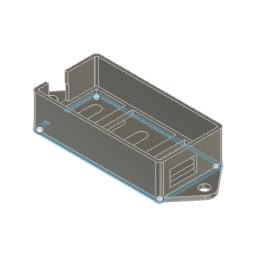
PSU case v4 (Autodesk Fusion 360 design; units mm, degrees)
Autodesk Fusion 360 part; units mm, degrees
sketch "Sketch1" plane through (0, 0, 0) normal (0, 0, 1) x (1, 0, 0) in component "card"
  line L0 (0, 0) -> (63, 0)
  line L1 (63, 0) -> (63, 30)
  line L2 (63, 30) -> (0, 30)
  line L3 (0, 30) -> (0, 0)
  line L4 (1, 29) -> (8.5, 29)
  line L5 (8.5, 29) -> (8.5, 19)
  line L6 (8.5, 19) -> (1, 19)
  line L7 (1, 19) -> (1, 29)
  line L8 (1, 6) -> (14.5, 6)
  line L9 (14.5, 6) -> (14.5, 15)
  line L10 (14.5, 15) -> (1, 15)
  line L11 (1, 15) -> (1, 6)
  line L12 (62, 29) -> (54.5, 29)
  line L13 (54.5, 29) -> (54.5, 19)
  line L14 (54.5, 19) -> (62, 19)
  line L15 (62, 19) -> (62, 29)
  line L16 (62, 4) -> (52, 4)
  line L17 (52, 4) -> (52, 17)
  line L18 (52, 17) -> (62, 17)
  line L19 (62, 17) -> (62, 4)
  dimension "d1" = 63
  dimension "d2" = 30
  dimension "d3" = 7.5
  dimension "d4" = 10
  dimension "d5" = 13.5
  dimension "d6" = 9
  dimension "d7" = 7.5
  dimension "d8" = 10
  dimension "d9" = 10
  dimension "d10" = 13
  constraint horizontal L0
  constraint vertical L1
  constraint horizontal L2
  constraint vertical L3
  constraint coincident L0.start L3.end
  constraint horizontal L4
  constraint vertical L5
  constraint horizontal L6
  constraint vertical L7
  constraint horizontal L8
  constraint vertical L9
  constraint horizontal L10
  constraint vertical L11
  constraint horizontal L12
  constraint vertical L13
  constraint horizontal L14
  constraint vertical L15
  constraint horizontal L16
  constraint vertical L17
  constraint horizontal L18
  constraint vertical L19
  measures "d1" distance of L0.start L0.end
  measures "d2" distance of L0.start L2.end
  measures "d3" distance of L4.start L4.end
  measures "d4" distance of L4.start L6.end
  measures "d5" distance of L8.start L8.end
  measures "d6" distance of L8.start L10.end
  measures "d7" distance of L12.start L12.end
  measures "d8" distance of L12.start L14.end
  measures "d9" distance of L16.start L16.end
  measures "d10" distance of L16.start L18.end
sketch "pcb support 0,4.5" plane through (0, 0, 0) normal (0, 0, 1) x (1, 0, 0) in component "bottom"
  line L0 (62.5, 29) -> (62.5, 1)
  line L1 (1, 1) -> (1, 29)
  line L2 (20, 1) -> (20, 29)
  line L3 (16.0721, 29) -> (16.0721, 1)
  line L4 (42.6148, 29) -> (42.6148, 1)
  line L5 (47, 1) -> (47, 29)
  line L6 (1, 29) -> (16.0721, 29)
  line L7 (20, 29) -> (42.6148, 29)
  line L8 (47, 29) -> (62.5, 29)
  line L9 (16.0721, 1) -> (1, 1)
  line L10 (62.5, 1) -> (47, 1)
  line L11 (42.6148, 1) -> (20, 1)
  line L12 (0, 32) -> (63, 32)
  line L13 (65, 30) -> (65, 0)
  line L14 (63, -2) -> (0, -2)
  line L15 (-2, 0) -> (-2, 30)
  arc A0 (0, 32) -> (-2, 30) centre (0, 30) ccw
  arc A1 (65, 30) -> (63, 32) centre (63, 30) ccw
  arc A2 (-2, 0) -> (0, -2) centre (0, 0) ccw
  arc A3 (63, -2) -> (65, 0) centre (63, 0) ccw
  dimension "d11" = 61.5
  dimension "d12" = 28
  dimension "d13" = 2
  constraint horizontal L6
  constraint vertical L0
  constraint horizontal L10
  constraint vertical L1
  constraint vertical L2
  constraint vertical L3
  constraint coincident L2.end L6
  constraint coincident L3.end L10
  constraint vertical L4
  constraint vertical L5
  constraint coincident L4.end L10
  constraint coincident L5.end L6
  constraint collinear L6 L7
  constraint collinear L7 L8
  constraint collinear L9 L10
  constraint collinear L10 L11
  constraint horizontal L12
  constraint vertical L13
  constraint horizontal L14
  constraint vertical L15
  constraint tangent L12 A0
  constraint tangent L15 A0
  constraint tangent L12 A1
  constraint tangent L13 A1
  constraint equal A0 A1
  constraint tangent L15 A2
  constraint tangent L14 A2
  constraint equal A0 A2
  constraint tangent L13 A3
  constraint tangent L14 A3
  constraint equal A0 A3
  measures "d11" distance of L1.end L0.start
  measures "d12" distance of L1.end L1.start
  measures "d13" radius of A0
sketch "bottom 0,2.0" plane through (0, 0, 0) normal (0, 0, 1) x (1, 0, 0) in component "bottom"
  line L0 (0, 32) -> (63, 32)
  arc A0 (64.5421, 31.2736) -> (63, 32) centre (63, 30) ccw
  arc A1 (63, -2) -> (64.4554, -1.3718) centre (63, 0) ccw
  line L1 (63, -2) -> (0, -2)
  arc A2 (-1.6548, -1.1232) -> (0, -2) centre (0, 0) ccw
  arc A3 (0, 32) -> (-1.6548, 31.1232) centre (0, 30) ccw
  circle A4 centre (-8.5, 15) radius 2.5
  circle A5 centre (71.5, 15) radius 2.5
  arc A6 (-12.2599, 18.2959) -> (-12.2599, 11.7041) centre (-8.5, 15) ccw
  arc A7 (75.2599, 11.7041) -> (75.2599, 18.2959) centre (71.5, 15) ccw
  line L2 (-12.2599, 18.2959) -> (-1.4142, 31.4142)
  line L3 (-12.2599, 11.7041) -> (-1.4142, -1.4142)
  line L4 (75.2599, 18.2959) -> (64.5421, 31.2736)
  line L5 (75.2599, 11.7041) -> (64.4554, -1.3718)
  dimension "d14" = 2
  dimension "d15" = 5
  dimension "d17" = 5
  dimension "d19" = 10
  dimension "d20" = 10
  constraint horizontal L0
  constraint horizontal L1
  constraint tangent L0 A3
  constraint tangent L0 A0
  constraint equal A0 A3
  constraint tangent L1 A2
  constraint equal A2 A3
  constraint tangent A1 L1
  constraint equal A1 A3
  constraint concentric A4 A6
  constraint concentric A5 A7
  constraint coincident L2 A3.end
  constraint coincident A3 L2.end
  constraint coincident L3 A2.start
  constraint coincident A2 L3.end
  constraint tangent A0 L4
  measures "d14" radius of A3
  measures "d15" diameter of A4
  measures "d17" diameter of A5
  measures "d19" diameter of A6
  measures "d20" diameter of A7
sketch "lower wall 0,12.5" plane through (0, 0, 0) normal (0, 0, 1) x (1, 0, 0) in component "bottom"
  line L0 (0.5, 30.5) -> (62.5, 30.5)
  line L1 (62.5, -0.5) -> (0.5, -0.5)
  line L2 (0, 32) -> (63, 32)
  arc A0 (0, 32) -> (-2, 30) centre (0, 30) ccw
  arc A1 (-2, 0) -> (0, -2) centre (0, 0) ccw
  line L3 (63, -2) -> (0, -2)
  arc A2 (63, -2) -> (65, 0) centre (63, 0) ccw
  arc A3 (65, 30) -> (63, 32) centre (63, 30) ccw
  arc A4 (0.5, 30.5) -> (-0.5, 29.5) centre (0.5, 29.5) ccw
  arc A5 (-0.5, 0.5) -> (0.5, -0.5) centre (0.5, 0.5) ccw
  arc A6 (63.5, 29.5) -> (62.5, 30.5) centre (62.5, 29.5) ccw
  arc A7 (62.5, -0.5) -> (63.5, 0.5) centre (62.5, 0.5) ccw
  line L4 (-2, 5) -> (-0.5, 5)
  line L5 (-2, 16) -> (-0.5, 16)
  line L6 (63.5, 3.5) -> (65, 3.5)
  line L7 (63.5, 17.5) -> (65, 17.5)
  line L8 (63.5, 29.5) -> (63.5, 17.5)
  line L9 (63.5, 3.5) -> (63.5, 0.5)
  line L10 (65, 30) -> (65, 17.5)
  line L11 (65, 3.5) -> (65, 0)
  line L12 (-2, 0) -> (-2, 5)
  line L13 (-2, 16) -> (-2, 30)
  line L14 (-0.5, 0.5) -> (-0.5, 5)
  line L15 (-0.5, 16) -> (-0.5, 29.5)
  dimension "d21" = 2
  dimension "d22" = 1
  dimension "d23" = 1
  dimension "d24" = 1
  dimension "d25" = 1
  constraint horizontal L0
  constraint vertical L8
  constraint horizontal L1
  constraint vertical L14
  constraint horizontal L2
  constraint vertical L10
  constraint horizontal L3
  constraint vertical L12
  constraint tangent L2 A0
  constraint tangent A0 L12
  constraint tangent L2 A3
  constraint tangent A3 L10
  constraint equal A0 A3
  constraint tangent A1 L12
  constraint tangent A1 L3
  constraint equal A0 A1
  constraint tangent A2 L10
  constraint tangent L3 A2
  constraint equal A0 A2
  constraint tangent L0 A4
  constraint tangent A4 L14
  constraint tangent A5 L14
  constraint tangent L1 A5
  constraint tangent L0 A6
  constraint tangent A6 L8
  constraint tangent A7 L8
  constraint tangent L1 A7
  constraint perpendicular L4 L14
  constraint coincident L5.start L12
  constraint coincident L5.end L14
  constraint perpendicular L5 L14
  constraint coincident L6.start L8
  constraint coincident L6.end L10
  constraint perpendicular L6 L10
  constraint perpendicular L7 L10
  constraint collinear L8 L9
  constraint collinear L10 L11
  constraint collinear L12 L13
  constraint collinear L14 L15
  measures "d21" radius of A0
  measures "d22" radius of A4
  measures "d23" radius of A5
  measures "d24" radius of A6
  measures "d25" radius of A7
sketch "upper wall 12.5/5.5" plane through (0, 0, 0) normal (0, 0, 1) x (1, 0, 0) in component "bottom"
  line L0 (-0.5, 16) -> (-0.5, 29.5)
  line L1 (-2, 0) -> (-2, 5)
  arc A0 (-0.5, 0.5) -> (0.5, -0.5) centre (0.5, 0.5) ccw
  line L2 (0.5, 30.5) -> (62.5, 30.5)
  line L3 (-0.5, 0.5) -> (-0.5, 5)
  line L4 (0, 32) -> (63, 32)
  arc A1 (0.5, 30.5) -> (-0.5, 29.5) centre (0.5, 29.5) ccw
  line L5 (-2, 16) -> (-2, 30)
  line L6 (62.5, -0.5) -> (0.5, -0.5)
  arc A2 (-2, 0) -> (0, -2) centre (0, 0) ccw
  arc A3 (0, 32) -> (-2, 30) centre (0, 30) ccw
  line L7 (63, -2) -> (0, -2)
  arc A4 (65, 30) -> (63, 32) centre (63, 30) ccw
  line L8 (65, 3.5) -> (65, 0)
  line L9 (63.5, 3.5) -> (63.5, 0.5)
  arc A5 (63, -2) -> (65, 0) centre (63, 0) ccw
  line L10 (63.5, 29.5) -> (63.5, 17.5)
  line L11 (65, 30) -> (65, 17.5)
  arc A6 (62.5, -0.5) -> (63.5, 0.5) centre (62.5, 0.5) ccw
  arc A7 (63.5, 29.5) -> (62.5, 30.5) centre (62.5, 29.5) ccw
  line L12 (63.5, 17.5) -> (63.5, 3.5)
  line L13 (65, 17.5) -> (65, 3.5)
  line L14 (-2, 15.5) -> (-0.5, 15.5)
  line L15 (-2, 5.5) -> (-0.5, 5.5)
  line L16 (-2, 5) -> (-2, 5.5)
  line L17 (-2, 15.5) -> (-2, 16)
  line L18 (-0.5, 16) -> (-0.5, 15.5)
  line L19 (-0.5, 5.5) -> (-0.5, 5)
  constraint perpendicular L14 L18
  constraint coincident L15.end L18
  constraint perpendicular L15 L18
  constraint coincident L14.start L16
  constraint collinear L16 L17
  constraint collinear L18 L19
extrude "Extrude1" add sketch "bottom 0,2.0" along normal blind 2 contours L0 A0 A1 L1 A2 A3 A6 A7 L2 L3 L4 L5 makes body 1
extrude "Extrude2" add sketch "pcb support 0,4.5" along normal blind 4.5 bodies 1
extrude "Extrude3" add sketch "lower wall 0,12.5" along normal blind 12.5 bodies 1
extrude "Extrude4" add sketch "upper wall 12.5/5.5" along normal blind 5.5 from surface at 12.5 bodies 1
sketch "top 0,1.5" plane through (0, 0, 0) normal (0, 0, 1) x (1, 0, 0) in component "top"
  line L0 (63, -2) -> (0, -2)
  line L1 (0, 32) -> (63, 32)
  line L2 (0, 32) -> (63, 32)
  line L3 (0, 32) -> (63, 32)
  line L4 (63, -2) -> (0, -2)
  line L5 (65, 30) -> (65, 17.5)
  line L6 (63, -2) -> (0, -2)
  line L7 (65, 30) -> (65, 0)
  arc A0 (63, -2) -> (65, 0) centre (63, 0) ccw
  line L8 (63, -2) -> (0, -2)
  arc A1 (63, -2) -> (65, 0) centre (63, 0) ccw
  arc A2 (65, 30) -> (63, 32) centre (63, 30) ccw
  arc A3 (63, -2) -> (64.4554, -1.3718) centre (63, 0) ccw
  arc A4 (65, 30) -> (63, 32) centre (63, 30) ccw
  arc A5 (0, 32) -> (-2, 30) centre (0, 30) ccw
  arc A6 (63, -2) -> (65, 0) centre (63, 0) ccw
  line L9 (0, 32) -> (63, 32)
  line L10 (65, 3.5) -> (65, 0)
  line L11 (65, 30) -> (65, 17.5)
  arc A7 (-1.6548, -1.1232) -> (0, -2) centre (0, 0) ccw
  arc A8 (64.5421, 31.2736) -> (63, 32) centre (63, 30) ccw
  line L12 (65, 3.5) -> (65, 0)
  arc A9 (65, 30) -> (63, 32) centre (63, 30) ccw
  line L13 (-2, 16) -> (-2, 30)
  arc A10 (-2, 0) -> (0, -2) centre (0, 0) ccw
  line L14 (-2, 16) -> (-2, 30)
  arc A11 (0, 32) -> (-1.6548, 31.1232) centre (0, 30) ccw
  line L15 (-2, 0) -> (-2, 30)
  arc A12 (0, 32) -> (-2, 30) centre (0, 30) ccw
  arc A13 (0, 32) -> (-2, 30) centre (0, 30) ccw
  arc A14 (-2, 0) -> (0, -2) centre (0, 0) ccw
  arc A15 (-2, 0) -> (0, -2) centre (0, 0) ccw
  line L16 (-2, 16) -> (-2, 5)
  line L17 (5, 22) -> (5, 8)
  line L18 (10, 22) -> (10, 8)
  arc A16 (10, 22) -> (5, 22) centre (7.5, 22) ccw
  arc A17 (5, 8) -> (10, 8) centre (7.5, 8) ccw
  line L19 (22, 22) -> (22, 8)
  arc A18 (22, 22) -> (17, 22) centre (19.5, 22) ccw
  arc A19 (17, 8) -> (22, 8) centre (19.5, 8) ccw
  line L20 (17, 22) -> (17, 8)
  line L21 (34, 22) -> (34, 8)
  arc A20 (34, 22) -> (29, 22) centre (31.5, 22) ccw
  arc A21 (29, 8) -> (34, 8) centre (31.5, 8) ccw
  line L22 (29, 22) -> (29, 8)
  line L23 (46, 22) -> (46, 8)
  arc A22 (46, 22) -> (41, 22) centre (43.5, 22) ccw
  arc A23 (41, 8) -> (46, 8) centre (43.5, 8) ccw
  line L24 (41, 22) -> (41, 8)
  line L25 (58, 22) -> (58, 8)
  arc A24 (58, 22) -> (53, 22) centre (55.5, 22) ccw
  arc A25 (53, 8) -> (58, 8) centre (55.5, 8) ccw
  line L26 (53, 22) -> (53, 8)
  point P0 (-1.4142, 31.4142)
  point P1 (-1.4142, -1.4142)
  dimension "d60" = 2
  dimension "d77" = 48
  dimension "d78" = 0
  constraint horizontal L9
  constraint vertical L5
  constraint horizontal L8
  constraint tangent L9 A12
  constraint tangent A2 L9
  constraint tangent L5 A2
  constraint equal A2 A12
  constraint tangent L8 A10
  constraint equal A10 A12
  constraint tangent L5 A6
  constraint tangent L8 A6
  constraint equal A6 A12
  constraint coincident L10.start L5
  constraint collinear L5 L10
  constraint vertical L17
  constraint perpendicular L1 L18
  constraint tangent L18 A16
  constraint tangent L17 A16
  constraint tangent L18 A17
  constraint tangent L17 A17
  measures "d60" radius of A12
sketch "lip 0,2.25" plane through (0, 0, 0) normal (0, 0, 1) x (1, 0, 0) in component "top"
  arc A0 (62.5, -0.35) -> (63.35, 0.5) centre (62.5, 0.5) ccw
  arc A1 (63.35, 29.5) -> (62.5, 30.35) centre (62.5, 29.5) ccw
  arc A2 (63.35, 29.5) -> (62.5, 30.35) centre (62.5, 29.5) ccw
  line L0 (63.35, 29.5) -> (63.35, 0.5)
  line L1 (63.35, 29.5) -> (63.35, 0.5)
  arc A3 (62.5, -0.35) -> (63.35, 0.5) centre (62.5, 0.5) ccw
  arc A4 (63.35, 29.5) -> (62.5, 30.35) centre (62.5, 29.5) ccw
  arc A5 (0.5, 30.35) -> (-0.35, 29.5) centre (0.5, 29.5) ccw
  line L2 (-0.35, 29.5) -> (-0.35, 0.5)
  line L3 (62.5, -0.35) -> (0.5, -0.35)
  line L4 (-0.35, 29.5) -> (-0.35, 0.5)
  arc A6 (-0.35, 0.5) -> (0.5, -0.35) centre (0.5, 0.5) ccw
  line L5 (0.5, 30.35) -> (62.5, 30.35)
  line L6 (62.5, -0.35) -> (0.5, -0.35)
  arc A7 (0.5, 30.35) -> (-0.35, 29.5) centre (0.5, 29.5) ccw
  line L7 (5, 22) -> (5, 8)
  arc A8 (29, 8) -> (34, 8) centre (31.5, 8) ccw
  line L8 (10, 22) -> (10, 8)
  arc A9 (34, 22) -> (29, 22) centre (31.5, 22) ccw
  arc A10 (10, 22) -> (5, 22) centre (7.5, 22) ccw
  line L9 (22, 22) -> (22, 8)
  line L10 (41, 22) -> (41, 8)
  arc A11 (46, 22) -> (41, 22) centre (43.5, 22) ccw
  arc A12 (5, 8) -> (10, 8) centre (7.5, 8) ccw
  line L11 (17, 22) -> (17, 8)
  arc A13 (58, 22) -> (53, 22) centre (55.5, 22) ccw
  arc A14 (22, 22) -> (17, 22) centre (19.5, 22) ccw
  arc A15 (17, 8) -> (22, 8) centre (19.5, 8) ccw
  line L12 (29, 22) -> (29, 8)
  arc A16 (41, 8) -> (46, 8) centre (43.5, 8) ccw
  arc A17 (53, 8) -> (58, 8) centre (55.5, 8) ccw
  line L13 (58, 22) -> (58, 8)
  line L14 (34, 22) -> (34, 8)
  line L15 (53, 22) -> (53, 8)
  line L16 (46, 22) -> (46, 8)
  point P0 (-1.4142, 31.4142)
  dimension "d81" = 48
  dimension "d82" = 0
  constraint tangent L1 A3
  constraint tangent A3 L3
  constraint tangent L3 A6
  constraint tangent L2 A7
  constraint tangent L2 A6
  constraint tangent A1 L1
  constraint tangent A5 L5
  constraint tangent A2 L5
  constraint tangent L0 A4
  constraint vertical L7
  constraint tangent L8 A10
  constraint tangent L7 A10
  constraint tangent L8 A12
  constraint tangent L7 A12
extrude "Extrude1'" add sketch "top 0,1.5" along normal blind 1.5 separate body makes body 2 in component "top"
extrude "Extrude2'" add sketch "lip 0,2.25" along normal blind 2.25 bodies 2 in component "top"
component "card" placed x (1, 0, 0) y (0, 1, 0) z (0, 0, 1) at (0, 0, 0)
component "bottom" placed x (1, 0, 0) y (0, 1, 0) z (0, 0, 1) at (0, 0, 0)
component "top" placed x (1, 0, 0) y (0, 1, 0) z (0, 0, 1) at (0, 0, 0)
